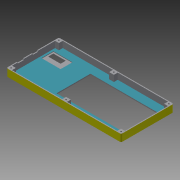
# Autodesk Inventor part: top-cover
Saved by Autodesk Inventor 2015 (Build 190159000, 159)
## iProperties
Created: 2016-04-26
Part Number: top-cover
Material: 一般
Document SubType Name: Modeling
Designer: yamashita1
Density: 1 g/cm^3
Appearance: 既定
Author: yamashita1
Autodesk Inventor part; units mm, degrees
ref_plane "YZ Plane" through (0, 0, 0) normal (1, 0, 0) x (0, 1, 0)
ref_plane "XZ Plane" through (0, 0, 0) normal (0, 1, 0) x (-1, 0, 0)
ref_plane "XY Plane" through (0, 0, 0) normal (0, 0, 1) x (1, 0, 0)
sketch "スケッチ1" plane through (0, 0, 0) normal (0, 0, 1) x (1, 0, 0)
  line L0 (-120, 55) -> (120, 55)
  line L1 (120, 55) -> (120, -55)
  line L2 (120, -55) -> (-120, -55)
  line L3 (-120, -55) -> (-120, 55)
  point P0 (0, 0)
  point P1 (0, -55)
  point P2 (120, 0)
  dimension "d0" = 240
  dimension "d1" = 110
  constraints: 8 end point, 2 midpoint, 2 parallel, 1 horizontal, 1 horizontal alignment, 1 perpendicular, 1 vertical alignment
  measures "d0" distance of L1.end L2.end
  measures "d1" distance of L0.end L1.end
extrude "天板" add sketch "スケッチ1" along normal blind 15
sketch "スケッチ2" plane through (0, 0, 15) normal (0, 0, 1) x (1, 0, 0)
  line L0 (-118, 53) -> (118, 53)
  line L1 (118, 53) -> (118, -53)
  line L2 (118, -53) -> (-118, -53)
  line L3 (-118, -53) -> (-118, 53)
  point P0 (0, 0)
  point P1 (0, -53)
  point P2 (118, 0)
  dimension "d4" = 236
  dimension "d5" = 106
  constraints: 8 end point, 2 midpoint, 2 parallel, 1 horizontal, 1 horizontal alignment, 1 perpendicular, 1 vertical alignment
  measures "d4" distance of L1.end L2.end
  measures "d5" distance of L2.end L0.start
extrude "天板くりぬき" cut sketch "スケッチ2" against normal blind 13
sketch "スケッチ3" plane through (0, 0, 2) normal (0, 0, 1) x (1, 0, 0)
  line L0 (-118, 53) -> (-110, 53)
  line L1 (-110, 53) -> (-110, 45)
  line L2 (-110, 45) -> (-118, 45)
  line L3 (-118, 45) -> (-118, 53)
  line L4 (-118, -45) -> (-110, -45)
  line L5 (-110, -45) -> (-110, -53)
  line L6 (-110, -53) -> (-118, -53)
  line L7 (-118, -53) -> (-118, -45)
  line L8 (110, 53) -> (118, 53)
  line L9 (118, 53) -> (118, 45)
  line L10 (118, 45) -> (110, 45)
  line L11 (110, 45) -> (110, 53)
  line L12 (110, -45) -> (118, -45)
  line L13 (118, -45) -> (118, -53)
  line L14 (118, -53) -> (110, -53)
  line L15 (110, -53) -> (110, -45)
  line L16 (-5, 53) -> (5, 53)
  line L17 (5, 53) -> (5, 45)
  line L18 (5, 45) -> (-5, 45)
  line L19 (-5, 45) -> (-5, 53)
  line L20 (-5, -45) -> (5, -45)
  line L21 (5, -45) -> (5, -53)
  line L22 (5, -53) -> (-5, -53)
  line L23 (-5, -53) -> (-5, -45)
  line L24 (-118, 53) -> (118, 53) projected
  line L25 (118, -53) -> (-118, -53) projected
  point P0 (0, 0)
  point P1 (0, 53)
  point P2 (0, 53)
  point P3 (0, -53)
  point P4 (0, -53)
  dimension "d8" = 8
  dimension "d9" = 8
  dimension "d10" = 10
  constraints: 48 end point, 12 parallel, 9 equal length, 6 coincident, 6 horizontal, 6 perpendicular, 4 midpoint, 2 collinear
  measures "d8" distance of L1.end L2.end
  measures "d9" distance of L0.end L1.end
  measures "d10" distance of L17.end L18.end
extrude "天板固定用ボス" add sketch "スケッチ3" along normal blind 13
sketch "スケッチ4" plane through (0, 0, 15) normal (0, 0, 1) x (1, 0, 0)
  circle A0 centre (-115, 50) radius 1.4
  circle A1 centre (-115, -50) radius 1.4
  circle A2 centre (0, -50) radius 1.4
  circle A3 centre (0, 50) radius 1.4
  circle A4 centre (115, 50) radius 1.4
  circle A5 centre (115, -50) radius 1.4
  line L0 (120, 55) -> (-120, 55) projected
  line L1 (-120, 55) -> (-120, -55) projected
  line L2 (-120, -55) -> (120, -55) projected
  line L3 (120, 55) -> (120, -55) projected
  point P0 (0, 0)
  dimension "d13" = 2.8
  dimension "d14" = 5
  dimension "d15" = 5
  dimension "d16" = 5
  dimension "d17" = 5
  constraints: 6 centre point, 5 equal radius, 5 horizontal alignment, 4 vertical alignment
  measures "d13" diameter of A0
  measures "d14" distance from line of L0 A0.centre
  measures "d15" distance from line of L1 A0.centre
  measures "d16" distance from line of L2 A1.centre
  measures "d17" distance from line of L3 A4.centre
extrude "天板固定用ねじ穴" cut sketch "スケッチ4" against normal blind 10 contours A0 | A1 | A2 | A3 | A4 | A5
sketch "スケッチ5" plane through (0, 0, 2) normal (0, 0, 1) x (1, 0, 0)
  line L0 (-34.5, 35.5) -> (110.5, 35.5)
  line L1 (110.5, 35.5) -> (110.5, -35.5)
  line L2 (110.5, -35.5) -> (-34.5, -35.5)
  line L3 (-34.5, -35.5) -> (-34.5, 35.5)
  line L4 (-85, 34.5) -> (-111, 34.5)
  line L5 (-111, 34.5) -> (-111, 23.5)
  line L6 (-111, 23.5) -> (-85, 23.5)
  line L7 (-85, 23.5) -> (-85, 34.5)
  point P0 (0, 0)
  point P1 (-10, 0)
  point P2 (86, 0)
  point P3 (38, 0)
  point P4 (38, 35.5)
  point P5 (-34.5, 0)
  point P6 (-85, 29)
  point P7 (-85, 29)
  dimension "d20" = 10
  dimension "d21" = 96
  dimension "d22" = 145
  dimension "d23" = 71
  dimension "d24" = 48
  dimension "d27" = 85
  dimension "d28" = 29
  dimension "d31" = 26
  dimension "d32" = 11
  constraints: 16 end point, 4 horizontal alignment, 4 parallel, 3 midpoint, 2 coincident, 2 horizontal, 2 perpendicular, 1 vertical alignment
  measures "d20" distance of point (-10, 0) point (0, 0)
  measures "d21" distance of point (86, 0) point (-10, 0)
  measures "d22" distance of L1.end L2.end
  measures "d23" distance of L0.end L1.end
  measures "d24" distance of point (38, 0) point (-10, 0)
  measures "d27" horizontal distance of point (-85, 29) point (0, 0)
  measures "d28" vertical distance of point (-85, 29) point (0, 0)
  measures "d31" distance of L6.end L5.end
  measures "d32" distance of L5.end L4.end
extrude "7セグ LCD用穴" cut sketch "スケッチ5" against normal blind 2
fillet "フィレット1" radius 3 4 edges at (120, -55, 7.5) (120, 55, 7.5) (-120, -55, 7.5) (-120, 55, 7.5)
sketch "スケッチ6" plane through (0, 0, 2) normal (0, 0, 1) x (1, 0, 0)
  line L0 (-114, 37.5) -> (-74, 37.5)
  line L1 (-74, 37.5) -> (-74, 12.5)
  line L2 (-74, 12.5) -> (-114, 12.5)
  line L3 (-114, 12.5) -> (-114, 37.5)
  line L4 (-85, 34.5) -> (-85, 23.5) projected
  line L5 (-111, 23.5) -> (-111, 34.5) projected
  point P0 (0, 0)
  point P1 (-74, 25)
  point P2 (-85, 29)
  dimension "d34" = 40
  dimension "d35" = 25
  dimension "d36" = 3
  dimension "d55" = 4
  constraints: 8 end point, 2 midpoint, 2 parallel, 1 horizontal, 1 perpendicular
  measures "d34" distance of L1.end L2.end
  measures "d35" distance of L0.end L1.end
  measures "d36" distance from line of L5 L2.end
  measures "d55" vertical distance of point (-85, 29) point (-74, 25)
extrude "LCD用くぼみ" cut sketch "スケッチ6" against normal blind 1.2
sketch "スケッチ8" plane through (-120, -52, 0) normal (-1, 0, 0) x (0, 0, 1)
  line L0 (0, 16.5) -> (0, 87.5) projected
  line L1 (15, 0) -> (15, 104) projected
  line L2 (15, 61.38) -> (13, 61.38)
  line L3 (13, 61.38) -> (13, 50.38)
  line L4 (13, 50.38) -> (15, 50.38)
  line L5 (15, 50.38) -> (15, 61.38)
  line L6 (15, 31.9) -> (13, 31.9)
  line L7 (13, 31.9) -> (13, 18.9)
  line L8 (13, 18.9) -> (15, 18.9)
  line L9 (15, 18.9) -> (15, 31.9)
  point P0 (0, 52)
  point P1 (0, 63.5)
  point P2 (15, 55.88)
  point P3 (15, 25.4)
  point P4 (15, 55.88)
  point P5 (15, 25.4)
  dimension "d46" = 11.5
  dimension "d47" = 7.62
  dimension "d48" = 38.1
  dimension "d49" = 2
  dimension "d50" = 11
  dimension "d51" = 2
  dimension "d52" = 13
  constraints: 16 end point, 4 parallel, 4 point on line, 3 coincident, 2 horizontal, 2 midpoint, 2 perpendicular
  measures "d46" distance of point (0, 52) point (0, 63.5)
  measures "d47" vertical distance of point (15, 55.88) point (0, 63.5)
  measures "d48" vertical distance of point (15, 25.4) point (0, 63.5)
  measures "d49" distance of L4.end L3.end
  measures "d50" distance of L3.end L2.end
  measures "d51" distance of L8.end L7.end
  measures "d52" distance of L7.end L6.end
extrude "Arduinoコネクタ穴" cut sketch "スケッチ8" against normal blind 2
